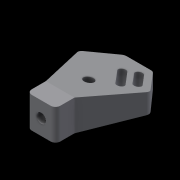
# Autodesk Inventor part: ForearmPistonConnector
Saved by Autodesk Inventor 2015 (Build 190159000, 159)
## iProperties
Created: 2014-11-15
Part Number: ForearmPistonConnector
Material: Generic
Document SubType Name: Modeling
Designer: Inventor
Mass: 0.841384 g
Surface Area: 8.25718 cm^2
Volume: 0.841384 cm^3
Density: 1 g/cm^3
Appearance: Default
Author: Inventor
Autodesk Inventor part; units mm, degrees
ref_plane "YZ Plane" through (0, 0, 0) normal (1, 0, 0) x (0, 1, 0)
ref_plane "XZ Plane" through (0, 0, 0) normal (0, 1, 0) x (-1, 0, 0)
sketch "Base" plane through (0, 0, 0) normal (0, 0, 1) x (1, 0, 0)
  line L0 (-7.5, 5.4092) -> (-3, 10.5)
  line L1 (-3, -6) -> (-3, -10)
  line L2 (-7.5, 5.4092) -> (-3, -6)
  line L3 (0, 10.5) -> (0, -10) construction
  line L4 (7.5, 5.4092) -> (3, 10.5)
  line L5 (3, -6) -> (3, -10)
  line L6 (7.5, 5.4092) -> (3, -6)
  circle A0 centre (0, 0) radius 1
  line L7 (0.5297, 6.5) -> (3.417, 3.2336) construction
  line L8 (2.5405, 8) -> (4.8181, 5.4233) construction
  circle A1 centre (0.5297, 6.5) radius 0.75
  circle A2 centre (2.5405, 8) radius 0.75
  circle A3 centre (3.417, 3.2336) radius 0.75
  circle A4 centre (4.8181, 5.4233) radius 0.75
  line L9 (-3, 10.5) -> (3, 10.5)
  line L10 (-3, -10) -> (3, -10)
  line L11 (3.1024, 8.4967) -> (5.3801, 5.92)
  line L12 (1.9786, 7.5033) -> (4.2562, 4.9266)
  line L13 (1.0917, 6.9967) -> (3.9789, 3.7303)
  line L14 (-0.0322, 6.0033) -> (2.8551, 2.7369)
  dimension "d13" = 2
  dimension "d14" = 1.5
  dimension "d17" = 2
  dimension "d18" = 2.5
  dimension "d20" = 6
  dimension "d23" = 117
  dimension "d24" = 6
  dimension "d25" = 15
  dimension "d26" = 4
  dimension "d28" = 2.5
  dimension "d29" = 3
  dimension "d30" = 2.5
  dimension "d31" = 4
  dimension "d32" = 16.5
  dimension "d56" = 10
  constraints: 30 end point, 8 point on circle, 7 tangent, 5 centre point, 5 coincident, 4 symmetric about line, 3 equal radius, 3 parallel, 2 horizontal, 2 midpoint, 1 perpendicular, 1 point on line, 1 vertical
  measures "d13" diameter of A0
  measures "d14" diameter of A1
  measures "d17" distance between parallel lines of L4 L8
  measures "d18" distance between parallel lines of L8 L7
  measures "d20" distance of L0.end L4.end
  measures "d23" angle of L2 L0
  measures "d24" distance of L1.end L5.end
  measures "d25" distance of L4.start L0.start
  measures "d26" distance of L1.start L1.end
  measures "d28" distance from line of L6 L8.end
  measures "d29" distance from line of L6 L7.end
  measures "d30" distance from line of L9 L8.start
  measures "d31" distance from line of L9 L7.start
  measures "d32" distance from line of L1.start L9
  measures "d56" distance from line of L10 A0.centre
extrude "BaseFeature" add sketch "Base" along normal blind 6.5
ref_plane "MidPlane" through (0, -13.6061, 0) normal (-1, 0, 0) x (0, 0, -1)
sketch "SideProfile" plane through (0, -13.6061, 0) normal (-1, 0, 0) x (0, 0, -1)
  line L0 (0, -24.1061) -> (-6.5, -24.1061) projected
  line L1 (-6.5, -7.6061) -> (-3, -24.1061)
  line L2 (-3, -24.1061) -> (0, -24.1061)
  line L3 (0, -24.1061) -> (0, -7.6061)
  line L4 (-6.5, -3.6061) -> (-6.5, -7.6061)
  line L5 (-6.5, -3.6061) -> (0, -3.6061)
  line L6 (0, -3.6061) -> (0, -7.6061)
  dimension "d37" = 3
  constraints: 12 end point, 2 horizontal, 1 perpendicular, 1 point on line, 1 vertical
  measures "d37" distance of L0.start L1.end
extrude "SideProfileFeature" cut sketch "SideProfile" along normal through all both and the other way through all keep common part
fillet "BaseFilletsFeature" radius 1 8 edges at (-3, 10.5, 1.5) (-7.5, 5.4092, 2.0399) (-3, -6, 3.25) (-3, -10, 3.25) (3, -10, 3.25) (3, -6, 3.25) (7.5, 5.4092, 2.0399) (3, 10.5, 1.5)
sketch "FrontHole" plane through (-2, -10, 6.5) normal (0, -1, 0) x (1, 0, 0)
  circle A0 centre (2, -3.25) radius 1.25
  line L0 (0, -6.5) -> (4, -6.5) projected
  line L1 (0, 0) -> (4, 0) projected
  line L2 (4, 0) -> (4, -6.5) projected
  line L3 (0, -6.5) -> (0, 0) projected
  dimension "d41" = 2.5
  dimension "d42" = 6.5
  dimension "d43" = 4
  dimension "d44" = 3.25
  dimension "d45" = 2
  constraints: 1 centre point
  measures "d41" diameter of A0
  measures "d42" distance between parallel lines of L0 L1
  measures "d43" distance between parallel lines of L2 L3
  measures "d44" distance from line of L1 A0.centre
  measures "d45" distance from line of L2 A0.centre
hole "FrontHoleFeature" at (0, -10, 3.25) direction (0, 1, 0) diameter 2 depth 6 tip angle 118
equation "\"d44\" = 0.5 * d42"
equation "\"d45\" = 0.5 * d43"
